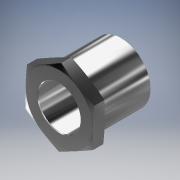
# Autodesk Inventor part: hex sleeve
Saved by Autodesk Inventor 2019 (Build 230136000, 136)
## iProperties
Shininess: 86.0
Length Units: 11272
Angle Units: 11279
Time Units: 11290
Mass Units: 11286
Length Display Precision: 3
Angle Display Precision: 2
Compacted: True
Created: 2001-07-10
Part Number: hex sleeve
Document SubType Name: Modeling
Designer: Autodesk, Inc.
Mass: 5.30137 g
Surface Area: 8.95541 cm^2
Volume: 0.65611 cm^3
Density: 8.08 g/cm^3
Material: Stainless Steel
Appearance: Chrome - Polished
Density: 0.0
Volumn: 0.0
Area: 0.0
PropertySet Name: Model Information
Control State: 0
Master: False
Checked Out: False
Author: Autodesk, Inc.
Autodesk Inventor part; units mm, degrees
ref_plane "YZ Plane" through (0, 0, 0) normal (1, 0, 0) x (0, 1, 0)
ref_plane "Work Plane1" through (0, 0, 0) normal (0, 0, 1) x (1, 0, 0)
sketch "Sketch2" plane through (0, 0, 0) normal (0, 0, 1) x (1, 0, 0)
  circle A0 centre (-0.5773, 0) radius 5.5562 projected
  circle A1 centre (-0.5773, 0) radius 3.9688
  dimension "d2" = 7.9375
  constraints: 1 centre point, 1 coincident
  measures "d2" diameter of A1
extrude "Extrusion1" add sketch "Sketch2" against normal blind 9.525
sketch "Sketch3" plane through (-0.5773, 0, 0) normal (0, 0, 1) x (1, 0, 0)
  line L0 (6.4585, 3.4714) -> (6.2356, -3.8575)
  line L1 (6.2356, -3.8575) -> (-0.2229, -7.329)
  line L2 (-0.2229, -7.329) -> (-6.4585, -3.4714)
  line L3 (-6.4585, -3.4714) -> (-6.2356, 3.8575)
  line L4 (-6.2356, 3.8575) -> (0.2229, 7.329)
  line L5 (0.2229, 7.329) -> (6.4585, 3.4714)
  circle A0 centre (0, 0) radius 3.9687 projected
  dimension "d5" = 12.7
  constraints: 12 end point, 11 other
  measures "d5" distance between parallel lines of L1 L4
extrude "Extrusion2" add sketch "Sketch3" along normal blind 2.286
chamfer "Chamfer1" distance 0.127 angle 45 3 edges at (-6.1335, 0, -9.525) (-4.546, 0, -9.525) (-4.546, 0, 2.286)
ref_plane "Work Plane2" through (-0.6887, -3.6645, 2.286) normal (0.9995, -0.0304, 0) x (0, 0, -1)
sketch "Sketch4" plane through (-0.6887, -3.6645, 2.286) normal (0.9995, -0.0304, 0) x (0, 0, -1)
  line L0 (0.127, 7.5779) -> (11.684, 7.5779) construction
  line L1 (0.0196, 8.031) -> (-0.0196, 11.6969) construction
  line L2 (2.286, 8.0308) -> (2.286, 11.697) construction
  line L3 (0, 9.8639) -> (0.6953, 13.8073)
  line L4 (0.6953, 13.8073) -> (0, 13.8073)
  line L5 (0, 13.8073) -> (0, 9.8639)
  line L6 (2.286, 9.8639) -> (2.286, 13.8395)
  line L7 (2.286, 13.8395) -> (1.585, 13.8395)
  line L8 (1.585, 13.8395) -> (2.286, 9.8639)
  line L9 (13.9688, 3.6092) -> (-4.4249, 3.6092)
  dimension "d11" = 10
  dimension "d12" = 2.286
  dimension "d13" = 10
  dimension "d14" = 2.286
  dimension "d15" = 3.9688
  constraints: 20 end point, 3 perpendicular, 2 midpoint, 2 parallel, 1 horizontal
  measures "d11" angle of L3 L5
  measures "d12" distance from line of L3.start L0
  measures "d13" angle of L8 L6
  measures "d14" distance from line of L6.start L0
  measures "d15" distance between parallel lines of L9 L0
revolve "Revolution1" cut sketch "Sketch4" angle 360 about axis through (-0.579, -0.057, -11.6828) along (0, 0, 1)
body "Solid1"
